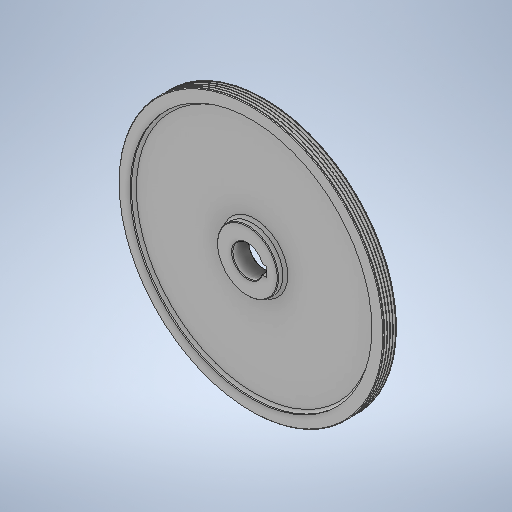
# Autodesk Inventor part: 29-10-203
Saved by Autodesk Inventor 2025.2 (Build 292293000, 293)
## iProperties
Created: 2024-11-29
Part Number: 29-10-203
Material: Generic
Document SubType Name: Modeling
Designer: Zvonko.Gabric
Density: 1 g/cm^3
Appearance: Default
Description: Polly-V pulley PJ4 11mm
Author: Zvonko.Gabric
Autodesk Inventor part; units mm, degrees
ref_plane "YZ Plane" through (0, 0, 0) normal (1, 0, 0) x (0, 1, 0)
ref_plane "XZ Plane" through (0, 0, 0) normal (0, 1, 0) x (-1, 0, 0)
ref_plane "XY Plane" through (0, 0, 0) normal (0, 0, 1) x (1, 0, 0)
sketch "Sketch1" plane through (0, 0, 0) normal (0, 1, 0) x (-1, 0, 0)
  line L0 (0, 11.1) -> (0, 0)
  line L1 (108.5, 10.6) -> (108, 11.1)
  line L2 (108.5, 10.0029) -> (108.5, 10.6)
  line L3 (106.5028, 9.2926) -> (108.5, 10.0029)
  line L4 (108.367, 7.9954) -> (106.5028, 8.6896)
  line L5 (106.5028, 6.9555) -> (108.367, 7.6186)
  line L6 (108.367, 5.6584) -> (106.5028, 6.3525)
  line L7 (106.5028, 4.6185) -> (108.367, 5.2815)
  line L8 (108.367, 3.3214) -> (106.5028, 4.0155)
  line L9 (106.5028, 2.2815) -> (108.367, 2.9445)
  line L10 (108.5, 0.9349) -> (106.5028, 1.6785)
  line L11 (108.5, 0.5) -> (108.5, 0.9349)
  line L12 (108, 0) -> (108.5, 0.5)
  line L13 (0, 0) -> (108, 0)
  line L14 (0, 11.1) -> (0, 0)
  line L15 (108, 11.1) -> (0, 11.1)
  arc A0 (106.5028, 9.2926) -> (106.5028, 8.6896) centre (106.61, 8.9911) ccw
  arc A1 (108.367, 7.6186) -> (108.367, 7.9954) centre (108.3, 7.807) ccw
  arc A2 (106.5028, 6.9555) -> (106.5028, 6.3525) centre (106.61, 6.654) ccw
  arc A3 (108.367, 5.2815) -> (108.367, 5.6584) centre (108.3, 5.47) ccw
  arc A4 (106.5028, 4.6185) -> (106.5028, 4.0155) centre (106.61, 4.317) ccw
  arc A5 (108.367, 2.9445) -> (108.367, 3.3214) centre (108.3, 3.133) ccw
  arc A6 (106.5028, 2.2815) -> (106.5028, 1.6785) centre (106.61, 1.98) ccw
  point P0 (108.5, 0.7174)
  point P1 (108.5, 10.3014)
  dimension "d0" = 0
  dimension "d1" = 11.1
  dimension "d2" = 108
  dimension "d3" = 0.7071
  dimension "d4" = 135
  dimension "d6" = 40
  dimension "d7" = 40
  dimension "d8" = 40
  dimension "d9" = 40
  dimension "d10" = 0.4349
  dimension "d11" = 135
  dimension "d12" = 135
  dimension "d13" = 135
  dimension "d14" = 108
  dimension "d15" = 108.5
  dimension "d16" = 2.109
  dimension "d17" = 3.293
  dimension "d18" = 4.446
  dimension "d19" = 5.63
  dimension "d20" = 6.783
  dimension "d21" = 7.967
  dimension "d22" = 9.12
  dimension "d23" = 1.89
  dimension "d24" = 0.2
  dimension "d25" = 1.89
  dimension "d26" = 0.2
  dimension "d27" = 0.2
  dimension "d28" = 1.89
  dimension "d29" = 0.2
  dimension "d30" = 1.89
  dimension "d31" = 0.32
  dimension "d32" = 0.2
  dimension "d33" = 0.32
  dimension "d34" = 0.2
  dimension "d35" = 0.32
  dimension "d36" = 0.2
  dimension "d37" = 0.32
  constraints: 32 end point, 14 point on circle, 7 centre point, 2 midpoint
  measures "d0" distance of point (0, 0) L0.end
  measures "d1" distance of L0.start L0.end
  measures "d2" distance of L1.end L0.start
  measures "d3" distance of L1.start L1.end
  measures "d4" angle of L2 L1
  measures "d6" angle of L4 L3
  measures "d7" angle of L6 L5
  measures "d8" angle of L8 L7
  measures "d9" angle of L10 L9
  measures "d10" distance of L11.start L10.start
  measures "d11" angle of L11 L12
  measures "d12" angle of L12 L13
  measures "d13" angle of L1 L15
  measures "d14" distance of L0.end L12.start
  measures "d15" distance from line of point (108.5, 0.717) L0
  measures "d16" distance from line of L15 A0.centre
  measures "d17" distance from line of L15 A1.centre
  measures "d18" distance from line of L15 A2.centre
  measures "d19" distance from line of L15 A3.centre
  measures "d20" distance from line of L15 A4.centre
  measures "d21" distance from line of L15 A5.centre
  measures "d22" distance from line of L15 A6.centre
  measures "d23" distance from line of L11 A6.centre
  measures "d24" distance from line of L11 A5.centre
  measures "d25" distance from line of L11 A4.centre
  measures "d26" distance from line of L11 A3.centre
  measures "d27" distance from line of L11 A1.centre
  measures "d28" horizontal distance of point (108.5, 0.717) A2.centre
  measures "d29" distance from line of L2 A1.centre
  measures "d30" horizontal distance of point (108.5, 10.301) A0.centre
  measures "d31" radius of A0
  measures "d32" radius of A1
  measures "d33" radius of A2
  measures "d34" radius of A3
  measures "d35" radius of A4
  measures "d36" radius of A5
  measures "d37" radius of A6
revolve "Revolution1" add sketch "Sketch1" angle 360 about axis through (0, 0, 11.1) along (0, 0, -1)
sketch "Sketch2" plane through (0, 0, 11.1) normal (0, 0, 1) x (1, 0, 0)
  circle A0 centre (0, 0) radius 99
  circle A1 centre (0, 0) radius 25
  dimension "d39" = 198
  dimension "d40" = 50
  constraints: 2 centre point, 2 coincident
  measures "d39" diameter of A0
  measures "d40" diameter of A1
extrude "Extrusion1" cut sketch "Sketch2" against normal blind 3.1
fillet "Fillet1" radius 2 2 edges at (-99, 0, 8) (-25, 0, 8)
sketch "Sketch3" plane through (0, 0, 0) normal (0, 0, -1) x (-1, 0, 0)
  arc A0 (-11.8427, -4) -> (-11.8427, 4) centre (0, 0) ccw
  line L0 (-12.5, 0) -> (-15.8, 0) construction
  line L1 (-15.8, 0) -> (-15.8, 4)
  line L2 (-15.8, 4) -> (-11.8427, 4)
  circle A1 centre (0, 0) radius 27 projected
  line L3 (-15.8, 0) -> (-15.8, -4)
  line L4 (-15.8, -4) -> (-11.8427, -4)
  point P0 (-8.0562, 4)
  point P1 (-8.0562, -4)
  point P2 (-13.8214, 4)
  dimension "d44" = 25
  dimension "d45" = 4
  dimension "d46" = 15.8
  dimension "d47" = 8
  dimension "d48" = 3.9573
  constraints: 10 end point, 2 perpendicular, 2 point on circle, 2 symmetric about line, 1 centre point, 1 coincident, 1 horizontal, 1 midpoint
  measures "d44" diameter of A0
  measures "d45" distance of L0.end L1.end
  measures "d46" distance from line of A1.centre L1
  measures "d47" distance from line of point (-13.821, 4) L4
  measures "d48" distance of L3.end L4.end
extrude "Extrusion2" cut sketch "Sketch3" along normal mid plane 100 contours L4 L3 L1 L2 A0
chamfer "Chamfer2" distance 0.5 angle 45 1 edges at (-12.5, 0, 0) measured on face at (-56.0076, -51.3382, 0)
fillet "Fillet2" radius 0.2 2 edges at (108.5, 0, 10.0029) (108.5, 0, 0.9349)
sketch "Sketch5" plane through (0, 0, 11.1) normal (0, 0, 1) x (1, 0, 0)
  circle A0 centre (0, 0) radius 25
  arc A1 (11.8427, 4) -> (11.8427, -4) centre (0, 0) ccw
  line L0 (15.8, -4) -> (11.8427, -4)
  line L1 (15.8, -4) -> (15.8, 4)
  line L2 (15.8, 4) -> (11.8427, 4)
  constraints: 6 end point, 2 centre point, 2 coincident, 2 point on circle, 1 horizontal, 1 perpendicular
extrude "Extrusion3" add sketch "Sketch5" along normal blind 2.9 contours A0 | L2 L1 L0 A1
sketch "Sketch6" plane through (0, 0, 11.1) normal (0, 0, -1) x (-1, 0, 0)
  arc A0 (-11.8427, -4) -> (-11.8427, 4) centre (0, 0) ccw
  line L0 (-15.8, -4) -> (-11.8427, -4)
  line L1 (-15.8, -4) -> (-15.8, 4) projected
  line L2 (-15.8, 4) -> (-11.8427, 4)
  line L3 (-15.8, 4) -> (-15.8, -4)
  constraints: 6 end point, 2 horizontal, 2 point on circle, 1 centre point, 1 coincident, 1 collinear
extrude "Extrusion4" cut sketch "Sketch6" against normal blind 100
chamfer "Chamfer3" distance 0.5 angle 45 2 edges at (-12.5, 0, 14) (-25, 0, 14) measured on face at (17.123, -11.6492, 14)
body "Solid1"
